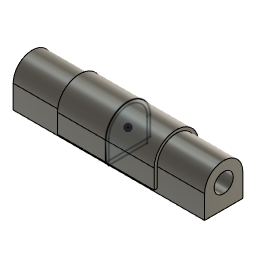
ClimbSim_HubParts v7 (Autodesk Fusion 360 design; units mm, degrees)
Autodesk Fusion 360 part; units mm, degrees
sketch "スケッチ4" plane through (0, 0, 0) normal (1, 0, 0) x (0, 1, 0)
  arc A0 (9.5, 0) -> (-9.5, 0) centre (0, 0) ccw
  line L0 (9.5, 0) -> (9.5, -11.5)
  line L1 (9.5, -11.5) -> (-9.5, -11.5)
  line L2 (-9.5, -11.5) -> (-9.5, 0)
  dimension "d8" = 9.5
  dimension "d9" = 19
  dimension "d10" = 11.5
  constraint coincident A0.centre origin
  constraint vertical L0
  constraint horizontal L1
  constraint vertical L2
  constraint coincident A0.start L0.start
  measures "d8" radius of A0
  measures "d9" distance of L0.end L1.end
  measures "d10" distance of A0.end L1
extrude "押し出し2" add sketch "スケッチ4" along normal mid plane 95
sketch "スケッチ6" plane through (0, 0, 0) normal (1, 0, 0) x (0, 1, 0)
  arc A0 (11, 0) -> (-11, 0) centre (0, 0) ccw
  line L0 (11, 0) -> (11, -9.5)
  line L1 (11, -9.5) -> (-11, -9.5)
  line L2 (-11, -9.5) -> (-11, 0)
  dimension "d17" = 9.5
  dimension "d18" = 22
  constraint coincident A0.centre origin
  constraint vertical L0
  constraint horizontal L1
  constraint vertical L2
  constraint coincident A0.start L0.start
  constraint equal L0 L2
  constraint tangent A0 L2
  measures "d17" distance of A0.start L0.end
  measures "d18" distance of L0.end L1.end
extrude "押し出し3" add sketch "スケッチ6" along normal mid plane 48
sketch "スケッチ7" plane through (47.5, 0, 0) normal (1, 0, 0) x (0, 1, 0)
  arc A0 (9.5, 0) -> (-9.5, 0) centre (0, 0) ccw
  line L0 (-9.5, 0) -> (-9.5, -11.5)
  line L1 (-9.5, -11.5) -> (9.5, -11.5)
  line L2 (9.5, -11.5) -> (9.5, 0)
  circle A1 centre (0, 0) radius 4.75
  dimension "d21" = 9.5
  constraint coincident A0.centre A1.centre
  measures "d21" diameter of A1
extrude "押し出し4" cut sketch "スケッチ7" along normal through all and the other way through all contours A1
